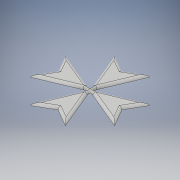
# Autodesk Inventor part: cross
Saved by Autodesk Inventor 2019 (Build 230136000, 136)
## iProperties
Created: 2023-02-19
Part Number: cross
Material: Generic
Document SubType Name: Modeling
Designer: Matt
Density: 1 g/cm^3
Appearance: Default
Author: Matt
Autodesk Inventor part; units mm, degrees
ref_plane "YZ Plane" through (0, 0, 0) normal (1, 0, 0) x (0, 1, 0)
ref_plane "XZ Plane" through (0, 0, 0) normal (0, 1, 0) x (-1, 0, 0)
ref_plane "XY Plane" through (0, 0, 0) normal (0, 0, 1) x (1, 0, 0)
sketch "Sketch1" plane through (0, 0, 0) normal (0, 1, 0) x (-1, 0, 0)
  line L0 (4, 0) -> (1.8224, 5.2573)
  line L1 (4, 0) -> (9.6904, 0) construction
  line L2 (4, 0) -> (6.1776, 5.2573)
  line L3 (4, 0) -> (9.6904, 0) construction
  line L4 (4, 0) -> (9.2573, 2.1776)
  line L5 (4, 0) -> (9.6904, 0) construction
  line L6 (4, 0) -> (9.2573, -2.1776)
  line L7 (4, 0) -> (9.6904, 0) construction
  line L8 (4, 0) -> (6.1776, -5.2573)
  line L9 (4, 0) -> (9.6904, 0) construction
  line L10 (4, 0) -> (1.8224, -5.2573)
  line L11 (4, 0) -> (9.6904, 0) construction
  line L12 (4, 0) -> (-1.2573, -2.1776)
  line L13 (4, 0) -> (9.6904, 0) construction
  line L14 (4, 0) -> (-1.2573, 2.1776)
  line L15 (4, 0) -> (9.6904, 0) construction
  line L16 (4, 4) -> (6.1776, 5.2573)
  line L17 (4, 4) -> (1.8224, 5.2573)
  line L18 (-1.2573, 2.1776) -> (0, 0)
  line L19 (0, 0) -> (-1.2573, -2.1776)
  line L20 (1.8224, -5.2573) -> (4, -4)
  line L21 (4, -4) -> (6.1776, -5.2573)
  line L22 (8, 0) -> (9.2573, -2.1776)
  line L23 (8, 0) -> (9.2573, 2.1776)
  dimension "d1" = 112.5
  dimension "d2" = 67.5
  dimension "d3" = 22.5
  dimension "d4" = 22.5
  dimension "d5" = 67.5
  dimension "d6" = 112.5
  dimension "d7" = 157.5
  dimension "d8" = 157.5
  constraints: 48 end point, 8 equal length, 8 horizontal, 6 perpendicular
  measures "d1" angle of L1 L0
  measures "d2" angle of L3 L2
  measures "d3" angle of L5 L4
  measures "d4" angle of L6 L7
  measures "d5" angle of L8 L9
  measures "d6" angle of L10 L11
  measures "d7" angle of L12 L13
  measures "d8" angle of L15 L14
extrude "Extrusion1" add sketch "Sketch1" along normal blind 2
sketch "Sketch2" plane through (0, 2, 0) normal (0, 1, 0) x (1, 0, 0)
  line L0 (-4, 0) -> (1.2573, -2.1776) projected
  line L1 (-1.8224, -5.2573) -> (-4, 0) projected
  line L2 (-9.2573, -2.1776) -> (-4, 0) projected
  line L3 (-4, 0) -> (-9.2573, 2.1776) projected
  line L4 (1.2573, 2.1776) -> (-4, 0) projected
  line L5 (-4, 0) -> (-1.8224, 5.2573) projected
  line L6 (-6.1776, 5.2573) -> (-4, 0) projected
  line L7 (-4, 0) -> (-6.1776, -5.2573) projected
  line L8 (-4.6, 0.2485) -> (-4, 0) construction
  line L9 (-4, 0) -> (-4.2485, 0.6) construction
  spline S0 degree 2 poles (-4.6, 0.2485) (-4, 0) (-4.2485, 0.6) knots 1 1 1 2 2 2
  line L10 (-3.4, 0.2485) -> (-4, 0) construction
  line L11 (-4, 0) -> (-3.7515, 0.6) construction
  spline S1 degree 2 poles (-3.4, 0.2485) (-4, 0) (-3.7515, 0.6) knots 1 1 1 2 2 2
  line L12 (-4.6, -0.2485) -> (-4, 0) construction
  line L13 (-4, 0) -> (-4.2485, -0.6) construction
  spline S2 degree 2 poles (-4.6, -0.2485) (-4, 0) (-4.2485, -0.6) knots 1 1 1 2 2 2
  line L14 (-3.7515, -0.6) -> (-4, 0) construction
  line L15 (-4, 0) -> (-3.4, -0.2485) construction
  spline S3 degree 2 poles (-3.7515, -0.6) (-4, 0) (-3.4, -0.2485) knots 1 1 1 2 2 2
  point P0 (0, 0)
  point P1 (-3.7, -0.1243)
  point P2 (-3.8757, -0.3)
  point P3 (-4.3, -0.1243)
  point P4 (-4.3, 0.1243)
  point P5 (-3.7, 0.1243)
  point P6 (-3.8757, 0.3)
  point P7 (-4.1243, 0.3)
  point P8 (-4.1243, -0.3)
  constraints: 16 point on line, 5 collinear, 4 coincident, 2 perpendicular, 12 other
extrude "Extrusion2" add sketch "Sketch2" against normal blind 2
fillet "Fillet3" radius 0.3 20 edges at (-8.6286, 2, 1.0888) (-8.6286, 2, -1.0888) (-4.2121, 2, -0.2121) (-5.2131, 2, -2.9286) (-6.9286, 2, -1.2131) (-4.2121, 2, 0.2121) (-5.2131, 2, 2.9286) (-6.9286, 2, 1.2131) (-3.7879, 2, 0.2121) (-1.0714, 2, 1.2131) (-2.7869, 2, 2.9286) (-2.9112, 2, 4.6286) (-5.0888, 2, 4.6286) (0.6286, 2, 1.0888) (0.6286, 2, -1.0888) (-3.7879, 2, -0.2121) (-2.7869, 2, -2.9286) (-1.0714, 2, -1.2131) (-2.9112, 2, -4.6286) (-5.0888, 2, -4.6286)
sketch "Sketch4" plane through (0, 0, 0) normal (0, -1, 0) x (1, 0, 0)
  line L0 (-11.3212, 5.7891) -> (4.4703, 5.7891)
  line L1 (4.4703, 5.7891) -> (4.4703, -6.2686)
  line L2 (4.4703, -6.2686) -> (-11.3212, -6.2686)
  line L3 (-11.3212, -6.2686) -> (-11.3212, 5.7891)
  point P0 (0, 0)
  constraints: 8 end point, 2 parallel, 1 horizontal, 1 perpendicular
extrude "Extrusion4" cut sketch "Sketch4" against normal blind 1.7
body "Solid1"
